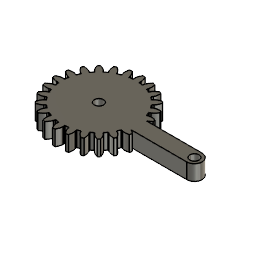
Simple gripper_Gear24 (Autodesk Fusion 360 design; units mm, degrees)
description: Spur Gear; Module: 1.125000; Num Teeth: 24; Pressure Angle: 20.000000; Backlash: 0.00 mm
Autodesk Fusion 360 part; units mm, degrees
(part 1 of 3)
sketch "Sketch4" plane through (0, 0, 3) normal (0, 0, 1) x (-1, 0, 0)
  arc A0 (-106.7629, 26.1027) -> (-106.8965, 25.0883) centre (-94.8448, 24.0176) ccw
  arc A1 (-107.004, 24.9974) -> (-106.8965, 25.0883) centre (-106.9961, 25.0971) ccw
  line L0 (-107.004, 24.9974) -> (-107.4897, 25.0359)
  spline S0 degree 5 poles (-107.4897, 25.0359) (-107.4953, 25.0363) (-107.5066, 25.0371) (-107.5235, 25.0378) (-107.5461, 25.0379) (-107.5744, 25.0371) (-107.6028, 25.0354) (-107.6311, 25.0332) (-107.6595, 25.0307) (-107.6879, 25.0281) (-107.7163, 25.0252) (-107.7447, 25.0221) (-107.7731, 25.0187) (-107.8015, 25.0149) (-107.83, 25.0108) (-107.8584, 25.0062) (-107.8868, 25.0014) (-107.9153, 24.9963) (-107.9437, 24.9909) (-107.9722, 24.9854) (-108.0006, 24.9796) (-108.029, 24.9736) (-108.0575, 24.9674) (-108.0859, 24.9609) (-108.1143, 24.9542) (-108.1428, 24.9473) (-108.1712, 24.9402) (-108.1996, 24.9328) (-108.228, 24.9252) (-108.2564, 24.9175) (-108.2848, 24.9095) (-108.3132, 24.9014) (-108.3416, 24.893) (-108.3699, 24.8845) (-108.3983, 24.8757) (-108.4266, 24.8668) (-108.455, 24.8577) (-108.4833, 24.8484) (-108.5116, 24.839) (-108.5399, 24.8293) (-108.5682, 24.8195) (-108.5965, 24.8095) (-108.6247, 24.7993) (-108.653, 24.789) (-108.6812, 24.7785) (-108.7094, 24.7678) (-108.7376, 24.7569) (-108.7658, 24.7459) (-108.794, 24.7347) (-108.8221, 24.7234) (-108.8503, 24.7119) (-108.8784, 24.7002) (-108.9065, 24.6884) (-108.9346, 24.6764) (-108.9627, 24.6643) (-108.9907, 24.652) (-109.0187, 24.6395) (-109.0467, 24.6269) (-109.0747, 24.6142) (-109.1027, 24.6013) (-109.1306, 24.5882) (-109.1586, 24.575) (-109.1865, 24.5616) (-109.2143, 24.5481) (-109.2422, 24.5345) (-109.27, 24.5207) (-109.2979, 24.5067) (-109.3256, 24.4927) (-109.3534, 24.4784) (-109.3811, 24.4641) (-109.4089, 24.4495) (-109.431, 24.4378) (-109.4476, 24.429) (-109.4587, 24.423) (-109.4642, 24.42) knots 0 0 0 0 0 0 0.01428571 0.02857143 0.04285714 0.05714286 0.07142857 0.08571429 0.1 0.11428571 0.12857143 0.14285714 0.15714286 0.17142857 0.18571429 0.2 0.21428571 0.22857143 0.24285714 0.25714286 0.27142857 0.28571429 0.3 0.31428571 0.32857143 0.34285714 0.35714286 0.37142857 0.38571429 0.4 0.41428571 0.42857143 0.44285714 0.45714286 0.47142857 0.48571429 0.5 0.51428571 0.52857143 0.54285714 0.55714286 0.57142857 0.58571429 0.6 0.61428571 0.62857143 0.64285714 0.65714286 0.67142857 0.68571429 0.7 0.71428571 0.72857143 0.74285714 0.75714286 0.77142857 0.78571429 0.8 0.81428571 0.82857143 0.84285714 0.85714286 0.87142857 0.88571429 0.9 0.91428571 0.92857143 0.94285714 0.95714286 0.97142857 0.98571429 1 1 1 1 1 1
  arc A2 (-109.4642, 24.42) -> (-109.4642, 23.6152) centre (-94.8448, 24.0176) ccw
  spline S1 degree 5 poles (-109.4642, 23.6152) (-109.4587, 23.6122) (-109.4476, 23.6062) (-109.431, 23.5974) (-109.4089, 23.5857) (-109.3811, 23.5712) (-109.3534, 23.5568) (-109.3256, 23.5425) (-109.2979, 23.5285) (-109.27, 23.5145) (-109.2422, 23.5007) (-109.2143, 23.4871) (-109.1865, 23.4736) (-109.1586, 23.4602) (-109.1306, 23.447) (-109.1027, 23.4339) (-109.0747, 23.421) (-109.0467, 23.4083) (-109.0187, 23.3957) (-108.9907, 23.3832) (-108.9627, 23.3709) (-108.9346, 23.3588) (-108.9065, 23.3468) (-108.8784, 23.335) (-108.8503, 23.3233) (-108.8221, 23.3118) (-108.794, 23.3005) (-108.7658, 23.2893) (-108.7376, 23.2783) (-108.7094, 23.2674) (-108.6812, 23.2568) (-108.653, 23.2462) (-108.6247, 23.2359) (-108.5965, 23.2257) (-108.5682, 23.2157) (-108.5399, 23.2059) (-108.5116, 23.1962) (-108.4833, 23.1868) (-108.455, 23.1775) (-108.4266, 23.1684) (-108.3983, 23.1595) (-108.3699, 23.1507) (-108.3416, 23.1422) (-108.3132, 23.1338) (-108.2848, 23.1257) (-108.2564, 23.1177) (-108.228, 23.11) (-108.1996, 23.1024) (-108.1712, 23.0951) (-108.1428, 23.0879) (-108.1143, 23.081) (-108.0859, 23.0743) (-108.0575, 23.0678) (-108.029, 23.0616) (-108.0006, 23.0556) (-107.9722, 23.0498) (-107.9437, 23.0443) (-107.9153, 23.0389) (-107.8868, 23.0338) (-107.8584, 23.029) (-107.83, 23.0244) (-107.8015, 23.0203) (-107.7731, 23.0165) (-107.7447, 23.0131) (-107.7163, 23.01) (-107.6879, 23.0071) (-107.6595, 23.0045) (-107.6311, 23.002) (-107.6028, 22.9998) (-107.5744, 22.9982) (-107.5461, 22.9973) (-107.5235, 22.9974) (-107.5066, 22.9981) (-107.4953, 22.9989) (-107.4897, 22.9993) knots -1 -1 -1 -1 -1 -1 -0.98571429 -0.97142857 -0.95714286 -0.94285714 -0.92857143 -0.91428571 -0.9 -0.88571429 -0.87142857 -0.85714286 -0.84285714 -0.82857143 -0.81428571 -0.8 -0.78571429 -0.77142857 -0.75714286 -0.74285714 -0.72857143 -0.71428571 -0.7 -0.68571429 -0.67142857 -0.65714286 -0.64285714 -0.62857143 -0.61428571 -0.6 -0.58571429 -0.57142857 -0.55714286 -0.54285714 -0.52857143 -0.51428571 -0.5 -0.48571429 -0.47142857 -0.45714286 -0.44285714 -0.42857143 -0.41428571 -0.4 -0.38571429 -0.37142857 -0.35714286 -0.34285714 -0.32857143 -0.31428571 -0.3 -0.28571429 -0.27142857 -0.25714286 -0.24285714 -0.22857143 -0.21428571 -0.2 -0.18571429 -0.17142857 -0.15714286 -0.14285714 -0.12857143 -0.11428571 -0.1 -0.08571429 -0.07142857 -0.05714286 -0.04285714 -0.02857143 -0.01428571 0 0 0 0 0 0
  line L1 (-107.4897, 22.9993) -> (-107.004, 23.0378)
  arc A3 (-106.8965, 22.947) -> (-107.004, 23.0378) centre (-106.9961, 22.9381) ccw
  arc A4 (-106.8965, 22.947) -> (-106.7629, 21.9326) centre (-94.8448, 24.0176) ccw
  arc A5 (-106.8433, 21.817) -> (-106.7629, 21.9326) centre (-106.8614, 21.9153) ccw
  line L2 (-106.8433, 21.817) -> (-107.3224, 21.7284)
  spline S2 degree 5 poles (-107.3224, 21.7284) (-107.3279, 21.7274) (-107.339, 21.7252) (-107.3556, 21.7215) (-107.3774, 21.7158) (-107.4045, 21.7076) (-107.4315, 21.6987) (-107.4583, 21.6892) (-107.4851, 21.6795) (-107.5118, 21.6696) (-107.5385, 21.6595) (-107.5651, 21.6492) (-107.5917, 21.6385) (-107.6182, 21.6275) (-107.6446, 21.6161) (-107.6709, 21.6044) (-107.6971, 21.5923) (-107.7232, 21.58) (-107.7493, 21.5675) (-107.7753, 21.5548) (-107.8013, 21.5418) (-107.8272, 21.5287) (-107.8531, 21.5153) (-107.8789, 21.5017) (-107.9046, 21.4879) (-107.9303, 21.4738) (-107.9559, 21.4596) (-107.9814, 21.4451) (-108.0069, 21.4305) (-108.0323, 21.4156) (-108.0577, 21.4006) (-108.083, 21.3854) (-108.1082, 21.37) (-108.1334, 21.3544) (-108.1586, 21.3386) (-108.1836, 21.3226) (-108.2086, 21.3065) (-108.2336, 21.2902) (-108.2585, 21.2737) (-108.2833, 21.2571) (-108.3081, 21.2403) (-108.3328, 21.2233) (-108.3575, 21.2062) (-108.3821, 21.1889) (-108.4067, 21.1714) (-108.4312, 21.1538) (-108.4556, 21.136) (-108.48, 21.118) (-108.5043, 21.1) (-108.5285, 21.0817) (-108.5527, 21.0633) (-108.5769, 21.0448) (-108.601, 21.0261) (-108.625, 21.0072) (-108.649, 20.9882) (-108.6729, 20.9691) (-108.6967, 20.9498) (-108.7205, 20.9304) (-108.7443, 20.9108) (-108.7679, 20.8911) (-108.7915, 20.8713) (-108.8151, 20.8513) (-108.8386, 20.8312) (-108.862, 20.8109) (-108.8854, 20.7905) (-108.9087, 20.77) (-108.932, 20.7493) (-108.9552, 20.7285) (-108.9783, 20.7076) (-109.0014, 20.6865) (-109.0244, 20.6654) (-109.0428, 20.6483) (-109.0565, 20.6354) (-109.0657, 20.6268) (-109.0702, 20.6225) knots 0 0 0 0 0 0 0.01428571 0.02857143 0.04285714 0.05714286 0.07142857 0.08571429 0.1 0.11428571 0.12857143 0.14285714 0.15714286 0.17142857 0.18571429 0.2 0.21428571 0.22857143 0.24285714 0.25714286 0.27142857 0.28571429 0.3 0.31428571 0.32857143 0.34285714 0.35714286 0.37142857 0.38571429 0.4 0.41428571 0.42857143 0.44285714 0.45714286 0.47142857 0.48571429 0.5 0.51428571 0.52857143 0.54285714 0.55714286 0.57142857 0.58571429 0.6 0.61428571 0.62857143 0.64285714 0.65714286 0.67142857 0.68571429 0.7 0.71428571 0.72857143 0.74285714 0.75714286 0.77142857 0.78571429 0.8 0.81428571 0.82857143 0.84285714 0.85714286 0.87142857 0.88571429 0.9 0.91428571 0.92857143 0.94285714 0.95714286 0.97142857 0.98571429 1 1 1 1 1 1
  arc A6 (-109.0702, 20.6225) -> (-108.8619, 19.8451) centre (-94.8448, 24.0176) ccw
  spline S3 degree 5 poles (-108.8619, 19.8451) (-108.8558, 19.8436) (-108.8436, 19.8408) (-108.8252, 19.8365) (-108.8008, 19.8309) (-108.7703, 19.8241) (-108.7398, 19.8174) (-108.7093, 19.8108) (-108.6788, 19.8044) (-108.6483, 19.7981) (-108.6178, 19.792) (-108.5874, 19.786) (-108.557, 19.7802) (-108.5266, 19.7745) (-108.4962, 19.769) (-108.4658, 19.7636) (-108.4354, 19.7584) (-108.4051, 19.7533) (-108.3748, 19.7484) (-108.3445, 19.7436) (-108.3142, 19.739) (-108.284, 19.7345) (-108.2538, 19.7302) (-108.2235, 19.7261) (-108.1934, 19.7221) (-108.1632, 19.7183) (-108.1331, 19.7146) (-108.103, 19.7111) (-108.0729, 19.7077) (-108.0428, 19.7046) (-108.0128, 19.7015) (-107.9828, 19.6987) (-107.9529, 19.696) (-107.9229, 19.6935) (-107.893, 19.6912) (-107.8632, 19.689) (-107.8333, 19.687) (-107.8035, 19.6852) (-107.7738, 19.6835) (-107.744, 19.6821) (-107.7144, 19.6808) (-107.6847, 19.6797) (-107.6551, 19.6788) (-107.6255, 19.6781) (-107.596, 19.6775) (-107.5665, 19.6772) (-107.5371, 19.6771) (-107.5077, 19.6771) (-107.4783, 19.6774) (-107.449, 19.6778) (-107.4198, 19.6785) (-107.3906, 19.6793) (-107.3614, 19.6805) (-107.3324, 19.6818) (-107.3033, 19.6834) (-107.2744, 19.6852) (-107.2455, 19.6872) (-107.2166, 19.6894) (-107.1878, 19.6918) (-107.1591, 19.6945) (-107.1305, 19.6975) (-107.1019, 19.7008) (-107.0735, 19.7045) (-107.0452, 19.7085) (-107.0169, 19.7129) (-106.9887, 19.7175) (-106.9606, 19.7223) (-106.9326, 19.7273) (-106.9046, 19.7325) (-106.8768, 19.7382) (-106.8493, 19.7447) (-106.8275, 19.7507) (-106.8113, 19.7557) (-106.8006, 19.7594) (-106.7953, 19.7613) knots -1 -1 -1 -1 -1 -1 -0.98571429 -0.97142857 -0.95714286 -0.94285714 -0.92857143 -0.91428571 -0.9 -0.88571429 -0.87142857 -0.85714286 -0.84285714 -0.82857143 -0.81428571 -0.8 -0.78571429 -0.77142857 -0.75714286 -0.74285714 -0.72857143 -0.71428571 -0.7 -0.68571429 -0.67142857 -0.65714286 -0.64285714 -0.62857143 -0.61428571 -0.6 -0.58571429 -0.57142857 -0.55714286 -0.54285714 -0.52857143 -0.51428571 -0.5 -0.48571429 -0.47142857 -0.45714286 -0.44285714 -0.42857143 -0.41428571 -0.4 -0.38571429 -0.37142857 -0.35714286 -0.34285714 -0.32857143 -0.31428571 -0.3 -0.28571429 -0.27142857 -0.25714286 -0.24285714 -0.22857143 -0.21428571 -0.2 -0.18571429 -0.17142857 -0.15714286 -0.14285714 -0.12857143 -0.11428571 -0.1 -0.08571429 -0.07142857 -0.05714286 -0.04285714 -0.02857143 -0.01428571 0 0 0 0 0 0
  line L3 (-106.7953, 19.7613) -> (-106.3361, 19.9241)
  arc A7 (-106.2087, 19.8642) -> (-106.3361, 19.9241) centre (-106.3027, 19.8299) ccw
  arc A8 (-106.2087, 19.8642) -> (-105.8172, 18.9189) centre (-94.8448, 24.0176) ccw
  arc A9 (-105.8649, 18.7865) -> (-105.8172, 18.9189) centre (-105.9079, 18.8768) ccw
  line L4 (-105.8649, 18.7865) -> (-106.3047, 18.577)
  spline S4 degree 5 poles (-106.3047, 18.577) (-106.3098, 18.5746) (-106.32, 18.5696) (-106.335, 18.5617) (-106.3546, 18.5505) (-106.3787, 18.5356) (-106.4024, 18.52) (-106.4259, 18.5039) (-106.4492, 18.4876) (-106.4725, 18.4711) (-106.4956, 18.4545) (-106.5187, 18.4376) (-106.5416, 18.4204) (-106.5643, 18.4029) (-106.5869, 18.3851) (-106.6092, 18.3669) (-106.6314, 18.3485) (-106.6535, 18.3299) (-106.6755, 18.311) (-106.6973, 18.292) (-106.7191, 18.2728) (-106.7407, 18.2534) (-106.7622, 18.2338) (-106.7836, 18.214) (-106.8049, 18.194) (-106.826, 18.1737) (-106.8471, 18.1533) (-106.868, 18.1328) (-106.8888, 18.112) (-106.9095, 18.0911) (-106.9301, 18.07) (-106.9506, 18.0487) (-106.971, 18.0273) (-106.9913, 18.0058) (-107.0115, 17.984) (-107.0316, 17.9621) (-107.0516, 17.9401) (-107.0715, 17.9178) (-107.0913, 17.8955) (-107.111, 17.873) (-107.1305, 17.8503) (-107.15, 17.8275) (-107.1694, 17.8046) (-107.1887, 17.7815) (-107.2079, 17.7583) (-107.227, 17.7349) (-107.246, 17.7114) (-107.2649, 17.6878) (-107.2837, 17.664) (-107.3024, 17.6401) (-107.321, 17.6161) (-107.3396, 17.5919) (-107.358, 17.5676) (-107.3763, 17.5432) (-107.3945, 17.5187) (-107.4127, 17.494) (-107.4307, 17.4692) (-107.4487, 17.4443) (-107.4666, 17.4193) (-107.4843, 17.3941) (-107.502, 17.3688) (-107.5196, 17.3434) (-107.5371, 17.3179) (-107.5544, 17.2923) (-107.5718, 17.2665) (-107.589, 17.2406) (-107.6061, 17.2147) (-107.6231, 17.1886) (-107.64, 17.1624) (-107.6569, 17.136) (-107.6736, 17.1096) (-107.6869, 17.0884) (-107.6969, 17.0724) (-107.7035, 17.0617) (-107.7068, 17.0564) knots 0 0 0 0 0 0 0.01428571 0.02857143 0.04285714 0.05714286 0.07142857 0.08571429 0.1 0.11428571 0.12857143 0.14285714 0.15714286 0.17142857 0.18571429 0.2 0.21428571 0.22857143 0.24285714 0.25714286 0.27142857 0.28571429 0.3 0.31428571 0.32857143 0.34285714 0.35714286 0.37142857 0.38571429 0.4 0.41428571 0.42857143 0.44285714 0.45714286 0.47142857 0.48571429 0.5 0.51428571 0.52857143 0.54285714 0.55714286 0.57142857 0.58571429 0.6 0.61428571 0.62857143 0.64285714 0.65714286 0.67142857 0.68571429 0.7 0.71428571 0.72857143 0.74285714 0.75714286 0.77142857 0.78571429 0.8 0.81428571 0.82857143 0.84285714 0.85714286 0.87142857 0.88571429 0.9 0.91428571 0.92857143 0.94285714 0.95714286 0.97142857 0.98571429 1 1 1 1 1 1
  arc A10 (-107.7068, 17.0564) -> (-107.3044, 16.3593) centre (-94.8448, 24.0176) ccw
  spline S5 degree 5 poles (-107.3044, 16.3593) (-107.2981, 16.3595) (-107.2855, 16.3599) (-107.2667, 16.3606) (-107.2417, 16.3615) (-107.2104, 16.3628) (-107.1792, 16.3642) (-107.148, 16.3657) (-107.1169, 16.3674) (-107.0859, 16.3693) (-107.0549, 16.3712) (-107.0239, 16.3734) (-106.993, 16.3756) (-106.9622, 16.378) (-106.9314, 16.3805) (-106.9007, 16.3832) (-106.87, 16.386) (-106.8394, 16.3889) (-106.8088, 16.392) (-106.7783, 16.3952) (-106.7479, 16.3986) (-106.7175, 16.4021) (-106.6872, 16.4058) (-106.6569, 16.4096) (-106.6268, 16.4136) (-106.5966, 16.4177) (-106.5666, 16.4219) (-106.5366, 16.4263) (-106.5067, 16.4309) (-106.4768, 16.4356) (-106.4471, 16.4405) (-106.4173, 16.4455) (-106.3877, 16.4506) (-106.3581, 16.456) (-106.3287, 16.4614) (-106.2993, 16.4671) (-106.2699, 16.4729) (-106.2407, 16.4788) (-106.2115, 16.4849) (-106.1824, 16.4912) (-106.1534, 16.4977) (-106.1245, 16.5043) (-106.0956, 16.5111) (-106.0669, 16.518) (-106.0382, 16.5252) (-106.0097, 16.5325) (-105.9812, 16.5399) (-105.9528, 16.5476) (-105.9245, 16.5554) (-105.8963, 16.5634) (-105.8682, 16.5717) (-105.8403, 16.5801) (-105.8124, 16.5887) (-105.7847, 16.5975) (-105.7571, 16.6066) (-105.7295, 16.6158) (-105.7021, 16.6252) (-105.6748, 16.6348) (-105.6477, 16.6446) (-105.6206, 16.6546) (-105.5937, 16.6649) (-105.567, 16.6755) (-105.5405, 16.6864) (-105.5142, 16.6977) (-105.488, 16.7092) (-105.462, 16.7209) (-105.4361, 16.7328) (-105.4103, 16.7449) (-105.3846, 16.7572) (-105.3593, 16.7699) (-105.3343, 16.7833) (-105.3148, 16.7947) (-105.3005, 16.8038) (-105.2911, 16.8101) (-105.2864, 16.8133) knots -1 -1 -1 -1 -1 -1 -0.98571429 -0.97142857 -0.95714286 -0.94285714 -0.92857143 -0.91428571 -0.9 -0.88571429 -0.87142857 -0.85714286 -0.84285714 -0.82857143 -0.81428571 -0.8 -0.78571429 -0.77142857 -0.75714286 -0.74285714 -0.72857143 -0.71428571 -0.7 -0.68571429 -0.67142857 -0.65714286 -0.64285714 -0.62857143 -0.61428571 -0.6 -0.58571429 -0.57142857 -0.55714286 -0.54285714 -0.52857143 -0.51428571 -0.5 -0.48571429 -0.47142857 -0.45714286 -0.44285714 -0.42857143 -0.41428571 -0.4 -0.38571429 -0.37142857 -0.35714286 -0.34285714 -0.32857143 -0.31428571 -0.3 -0.28571429 -0.27142857 -0.25714286 -0.24285714 -0.22857143 -0.21428571 -0.2 -0.18571429 -0.17142857 -0.15714286 -0.14285714 -0.12857143 -0.11428571 -0.1 -0.08571429 -0.07142857 -0.05714286 -0.04285714 -0.02857143 -0.01428571 0 0 0 0 0 0
  line L5 (-105.2864, 16.8133) -> (-104.8851, 17.0894)
  arc A11 (-104.7465, 17.0645) -> (-104.8851, 17.0894) centre (-104.8284, 17.0071) ccw
  arc A12 (-104.7465, 17.0645) -> (-104.1237, 16.2528) centre (-94.8448, 24.0176) ccw
  arc A13 (-104.1355, 16.1126) -> (-104.1237, 16.2528) centre (-104.2004, 16.1886) ccw
  line L6 (-104.1355, 16.1126) -> (-104.5061, 15.7963)
  spline S6 degree 5 poles (-104.5061, 15.7963) (-104.5104, 15.7926) (-104.5189, 15.7852) (-104.5314, 15.7737) (-104.5475, 15.7579) (-104.5669, 15.7372) (-104.5857, 15.716) (-104.6042, 15.6944) (-104.6225, 15.6726) (-104.6407, 15.6506) (-104.6588, 15.6286) (-104.6767, 15.6063) (-104.6944, 15.5838) (-104.7118, 15.561) (-104.729, 15.5379) (-104.7459, 15.5146) (-104.7625, 15.4911) (-104.779, 15.4674) (-104.7954, 15.4435) (-104.8116, 15.4194) (-104.8276, 15.3952) (-104.8435, 15.3709) (-104.8592, 15.3464) (-104.8747, 15.3217) (-104.8901, 15.2969) (-104.9053, 15.2719) (-104.9203, 15.2467) (-104.9352, 15.2214) (-104.9499, 15.196) (-104.9645, 15.1704) (-104.979, 15.1447) (-104.9933, 15.1189) (-105.0075, 15.0929) (-105.0215, 15.0668) (-105.0353, 15.0406) (-105.0491, 15.0143) (-105.0627, 14.9878) (-105.0761, 14.9612) (-105.0895, 14.9345) (-105.1027, 14.9076) (-105.1157, 14.8807) (-105.1286, 14.8536) (-105.1414, 14.8264) (-105.1541, 14.7992) (-105.1666, 14.7718) (-105.179, 14.7442) (-105.1913, 14.7166) (-105.2034, 14.6889) (-105.2154, 14.6611) (-105.2273, 14.6332) (-105.2391, 14.6051) (-105.2507, 14.577) (-105.2622, 14.5488) (-105.2736, 14.5204) (-105.2849, 14.492) (-105.296, 14.4635) (-105.307, 14.4348) (-105.3179, 14.4061) (-105.3287, 14.3773) (-105.3393, 14.3484) (-105.3499, 14.3194) (-105.3603, 14.2903) (-105.3706, 14.2612) (-105.3807, 14.2319) (-105.3908, 14.2026) (-105.4007, 14.1731) (-105.4105, 14.1436) (-105.4202, 14.114) (-105.4298, 14.0843) (-105.4392, 14.0545) (-105.4486, 14.0246) (-105.4559, 14.0007) (-105.4614, 13.9827) (-105.465, 13.9707) (-105.4668, 13.9647) knots 0 0 0 0 0 0 0.01428571 0.02857143 0.04285714 0.05714286 0.07142857 0.08571429 0.1 0.11428571 0.12857143 0.14285714 0.15714286 0.17142857 0.18571429 0.2 0.21428571 0.22857143 0.24285714 0.25714286 0.27142857 0.28571429 0.3 0.31428571 0.32857143 0.34285714 0.35714286 0.37142857 0.38571429 0.4 0.41428571 0.42857143 0.44285714 0.45714286 0.47142857 0.48571429 0.5 0.51428571 0.52857143 0.54285714 0.55714286 0.57142857 0.58571429 0.6 0.61428571 0.62857143 0.64285714 0.65714286 0.67142857 0.68571429 0.7 0.71428571 0.72857143 0.74285714 0.75714286 0.77142857 0.78571429 0.8 0.81428571 0.82857143 0.84285714 0.85714286 0.87142857 0.88571429 0.9 0.91428571 0.92857143 0.94285714 0.95714286 0.97142857 0.98571429 1 1 1 1 1 1
  arc A14 (-105.4668, 13.9647) -> (-104.8977, 13.3955) centre (-94.8448, 24.0176) ccw
  spline S7 degree 5 poles (-104.8977, 13.3955) (-104.8917, 13.3973) (-104.8797, 13.4009) (-104.8617, 13.4064) (-104.8377, 13.4138) (-104.8078, 13.4231) (-104.7781, 13.4326) (-104.7484, 13.4422) (-104.7188, 13.4518) (-104.6892, 13.4617) (-104.6598, 13.4716) (-104.6304, 13.4816) (-104.6012, 13.4918) (-104.572, 13.5021) (-104.5429, 13.5125) (-104.5139, 13.523) (-104.485, 13.5337) (-104.4562, 13.5444) (-104.4275, 13.5553) (-104.3989, 13.5663) (-104.3704, 13.5775) (-104.3419, 13.5887) (-104.3136, 13.6001) (-104.2854, 13.6116) (-104.2572, 13.6233) (-104.2292, 13.635) (-104.2013, 13.6469) (-104.1734, 13.6589) (-104.1457, 13.6711) (-104.1181, 13.6833) (-104.0906, 13.6957) (-104.0632, 13.7083) (-104.0359, 13.7209) (-104.0087, 13.7337) (-103.9817, 13.7466) (-103.9547, 13.7597) (-103.9279, 13.7729) (-103.9012, 13.7862) (-103.8746, 13.7997) (-103.8481, 13.8133) (-103.8217, 13.827) (-103.7955, 13.8409) (-103.7694, 13.8549) (-103.7435, 13.8691) (-103.7176, 13.8834) (-103.6919, 13.8978) (-103.6664, 13.9124) (-103.6409, 13.9272) (-103.6156, 13.942) (-103.5905, 13.9571) (-103.5655, 13.9723) (-103.5406, 13.9876) (-103.516, 14.0032) (-103.4914, 14.0189) (-103.4671, 14.0348) (-103.4429, 14.0508) (-103.4189, 14.067) (-103.395, 14.0833) (-103.3713, 14.0998) (-103.3477, 14.1165) (-103.3244, 14.1334) (-103.3014, 14.1505) (-103.2786, 14.168) (-103.2561, 14.1856) (-103.2338, 14.2035) (-103.2117, 14.2216) (-103.1898, 14.2398) (-103.168, 14.2581) (-103.1464, 14.2767) (-103.1251, 14.2955) (-103.1045, 14.3149) (-103.0886, 14.331) (-103.0772, 14.3435) (-103.0697, 14.352) (-103.066, 14.3563) knots -1 -1 -1 -1 -1 -1 -0.98571429 -0.97142857 -0.95714286 -0.94285714 -0.92857143 -0.91428571 -0.9 -0.88571429 -0.87142857 -0.85714286 -0.84285714 -0.82857143 -0.81428571 -0.8 -0.78571429 -0.77142857 -0.75714286 -0.74285714 -0.72857143 -0.71428571 -0.7 -0.68571429 -0.67142857 -0.65714286 -0.64285714 -0.62857143 -0.61428571 -0.6 -0.58571429 -0.57142857 -0.55714286 -0.54285714 -0.52857143 -0.51428571 -0.5 -0.48571429 -0.47142857 -0.45714286 -0.44285714 -0.42857143 -0.41428571 -0.4 -0.38571429 -0.37142857 -0.35714286 -0.34285714 -0.32857143 -0.31428571 -0.3 -0.28571429 -0.27142857 -0.25714286 -0.24285714 -0.22857143 -0.21428571 -0.2 -0.18571429 -0.17142857 -0.15714286 -0.14285714 -0.12857143 -0.11428571 -0.1 -0.08571429 -0.07142857 -0.05714286 -0.04285714 -0.02857143 -0.01428571 0 0 0 0 0 0
  line L7 (-103.066, 14.3563) -> (-102.7498, 14.7269)
  arc A15 (-102.6096, 14.7387) -> (-102.7498, 14.7269) centre (-102.6737, 14.662) ccw
  arc A16 (-102.6096, 14.7387) -> (-101.7978, 14.1158) centre (-94.8448, 24.0176) ccw
  arc A17 (-101.7729, 13.9773) -> (-101.7978, 14.1158) centre (-101.8553, 14.034) ccw
  line L8 (-101.7729, 13.9773) -> (-102.0491, 13.5759)
  spline S8 degree 5 poles (-102.0491, 13.5759) (-102.0523, 13.5713) (-102.0586, 13.5619) (-102.0676, 13.5475) (-102.0791, 13.528) (-102.0925, 13.5031) (-102.1052, 13.4777) (-102.1175, 13.4521) (-102.1295, 13.4263) (-102.1414, 13.4004) (-102.1532, 13.3743) (-102.1647, 13.3482) (-102.1759, 13.3219) (-102.1869, 13.2954) (-102.1975, 13.2686) (-102.2077, 13.2418) (-102.2178, 13.2147) (-102.2276, 13.1875) (-102.2372, 13.1602) (-102.2466, 13.1328) (-102.2558, 13.1053) (-102.2648, 13.0777) (-102.2737, 13.0499) (-102.2823, 13.0221) (-102.2907, 12.9941) (-102.2989, 12.966) (-102.3069, 12.9378) (-102.3148, 12.9096) (-102.3224, 12.8812) (-102.3299, 12.8527) (-102.3372, 12.8241) (-102.3443, 12.7955) (-102.3513, 12.7667) (-102.3581, 12.7379) (-102.3647, 12.709) (-102.3711, 12.68) (-102.3774, 12.6509) (-102.3835, 12.6217) (-102.3895, 12.5924) (-102.3953, 12.5631) (-102.4009, 12.5337) (-102.4064, 12.5042) (-102.4117, 12.4746) (-102.4169, 12.445) (-102.4219, 12.4153) (-102.4268, 12.3855) (-102.4315, 12.3557) (-102.436, 12.3258) (-102.4404, 12.2958) (-102.4447, 12.2657) (-102.4488, 12.2356) (-102.4527, 12.2054) (-102.4565, 12.1752) (-102.4602, 12.1448) (-102.4637, 12.1145) (-102.4671, 12.084) (-102.4703, 12.0535) (-102.4734, 12.023) (-102.4764, 11.9924) (-102.4792, 11.9617) (-102.4818, 11.931) (-102.4844, 11.9002) (-102.4868, 11.8693) (-102.489, 11.8384) (-102.4911, 11.8075) (-102.4931, 11.7765) (-102.4949, 11.7454) (-102.4966, 11.7143) (-102.4982, 11.6832) (-102.4996, 11.6519) (-102.5009, 11.6207) (-102.5018, 11.5956) (-102.5024, 11.5768) (-102.5028, 11.5643) (-102.503, 11.558) knots 0 0 0 0 0 0 0.01428571 0.02857143 0.04285714 0.05714286 0.07142857 0.08571429 0.1 0.11428571 0.12857143 0.14285714 0.15714286 0.17142857 0.18571429 0.2 0.21428571 0.22857143 0.24285714 0.25714286 0.27142857 0.28571429 0.3 0.31428571 0.32857143 0.34285714 0.35714286 0.37142857 0.38571429 0.4 0.41428571 0.42857143 0.44285714 0.45714286 0.47142857 0.48571429 0.5 0.51428571 0.52857143 0.54285714 0.55714286 0.57142857 0.58571429 0.6 0.61428571 0.62857143 0.64285714 0.65714286 0.67142857 0.68571429 0.7 0.71428571 0.72857143 0.74285714 0.75714286 0.77142857 0.78571429 0.8 0.81428571 0.82857143 0.84285714 0.85714286 0.87142857 0.88571429 0.9 0.91428571 0.92857143 0.94285714 0.95714286 0.97142857 0.98571429 1 1 1 1 1 1
  arc A18 (-102.503, 11.558) -> (-101.806, 11.1556) centre (-94.8448, 24.0176) ccw
  spline S9 degree 5 poles (-101.806, 11.1556) (-101.8006, 11.1589) (-101.7899, 11.1655) (-101.774, 11.1754) (-101.7527, 11.1887) (-101.7263, 11.2055) (-101.7, 11.2223) (-101.6738, 11.2393) (-101.6477, 11.2563) (-101.6217, 11.2734) (-101.5958, 11.2906) (-101.5701, 11.3079) (-101.5445, 11.3253) (-101.5189, 11.3428) (-101.4935, 11.3604) (-101.4683, 11.378) (-101.4431, 11.3958) (-101.4181, 11.4137) (-101.3931, 11.4316) (-101.3683, 11.4497) (-101.3437, 11.4678) (-101.3191, 11.486) (-101.2947, 11.5044) (-101.2704, 11.5228) (-101.2463, 11.5413) (-101.2222, 11.5599) (-101.1983, 11.5786) (-101.1746, 11.5975) (-101.1509, 11.6164) (-101.1274, 11.6354) (-101.1041, 11.6545) (-101.0808, 11.6736) (-101.0578, 11.6929) (-101.0348, 11.7123) (-101.012, 11.7318) (-100.9894, 11.7514) (-100.9669, 11.7711) (-100.9445, 11.7909) (-100.9223, 11.8108) (-100.9002, 11.8307) (-100.8783, 11.8508) (-100.8566, 11.871) (-100.835, 11.8913) (-100.8136, 11.9117) (-100.7924, 11.9322) (-100.7713, 11.9528) (-100.7504, 11.9735) (-100.7296, 11.9944) (-100.709, 12.0153) (-100.6886, 12.0363) (-100.6684, 12.0575) (-100.6484, 12.0788) (-100.6286, 12.1001) (-100.609, 12.1217) (-100.5896, 12.1433) (-100.5703, 12.165) (-100.5513, 12.1869) (-100.5325, 12.2089) (-100.5138, 12.2309) (-100.4954, 12.2531) (-100.4773, 12.2755) (-100.4594, 12.298) (-100.4419, 12.3207) (-100.4248, 12.3436) (-100.4079, 12.3667) (-100.3912, 12.3899) (-100.3747, 12.4131) (-100.3584, 12.4365) (-100.3423, 12.4599) (-100.3267, 12.4836) (-100.3118, 12.5077) (-100.3006, 12.5274) (-100.2928, 12.5424) (-100.2878, 12.5525) (-100.2854, 12.5577) knots -1 -1 -1 -1 -1 -1 -0.98571429 -0.97142857 -0.95714286 -0.94285714 -0.92857143 -0.91428571 -0.9 -0.88571429 -0.87142857 -0.85714286 -0.84285714 -0.82857143 -0.81428571 -0.8 -0.78571429 -0.77142857 -0.75714286 -0.74285714 -0.72857143 -0.71428571 -0.7 -0.68571429 -0.67142857 -0.65714286 -0.64285714 -0.62857143 -0.61428571 -0.6 -0.58571429 -0.57142857 -0.55714286 -0.54285714 -0.52857143 -0.51428571 -0.5 -0.48571429 -0.47142857 -0.45714286 -0.44285714 -0.42857143 -0.41428571 -0.4 -0.38571429 -0.37142857 -0.35714286 -0.34285714 -0.32857143 -0.31428571 -0.3 -0.28571429 -0.27142857 -0.25714286 -0.24285714 -0.22857143 -0.21428571 -0.2 -0.18571429 -0.17142857 -0.15714286 -0.14285714 -0.12857143 -0.11428571 -0.1 -0.08571429 -0.07142857 -0.05714286 -0.04285714 -0.02857143 -0.01428571 0 0 0 0 0 0
  line L9 (-100.2854, 12.5577) -> (-100.0758, 12.9975)
  arc A19 (-99.9434, 13.0452) -> (-100.0758, 12.9975) centre (-99.9856, 12.9545) ccw
  arc A20 (-99.9434, 13.0452) -> (-98.9981, 12.6536) centre (-94.8448, 24.0176) ccw
  arc A21 (-98.9382, 12.5263) -> (-98.9981, 12.6536) centre (-99.0325, 12.5597) ccw
  line L10 (-98.9382, 12.5263) -> (-99.1011, 12.0671)
  spline S10 degree 5 poles (-99.1011, 12.0671) (-99.103, 12.0618) (-99.1066, 12.0511) (-99.1117, 12.0349) (-99.1177, 12.0131) (-99.1242, 11.9855) (-99.1299, 11.9577) (-99.1351, 11.9298) (-99.1401, 11.9017) (-99.1448, 11.8736) (-99.1494, 11.8454) (-99.1538, 11.8172) (-99.1579, 11.7889) (-99.1616, 11.7604) (-99.1649, 11.7319) (-99.1679, 11.7032) (-99.1705, 11.6745) (-99.173, 11.6457) (-99.1752, 11.6169) (-99.1772, 11.588) (-99.179, 11.559) (-99.1805, 11.53) (-99.1819, 11.5009) (-99.183, 11.4718) (-99.1839, 11.4426) (-99.1846, 11.4133) (-99.185, 11.384) (-99.1852, 11.3547) (-99.1853, 11.3253) (-99.1851, 11.2958) (-99.1848, 11.2664) (-99.1843, 11.2368) (-99.1836, 11.2073) (-99.1827, 11.1776) (-99.1816, 11.148) (-99.1803, 11.1183) (-99.1788, 11.0886) (-99.1772, 11.0588) (-99.1754, 11.029) (-99.1734, 10.9992) (-99.1712, 10.9693) (-99.1689, 10.9394) (-99.1663, 10.9095) (-99.1637, 10.8795) (-99.1608, 10.8495) (-99.1578, 10.8195) (-99.1546, 10.7895) (-99.1513, 10.7594) (-99.1478, 10.7293) (-99.1441, 10.6991) (-99.1403, 10.669) (-99.1363, 10.6388) (-99.1321, 10.6086) (-99.1278, 10.5784) (-99.1234, 10.5481) (-99.1187, 10.5178) (-99.114, 10.4876) (-99.1091, 10.4572) (-99.104, 10.4269) (-99.0987, 10.3966) (-99.0934, 10.3662) (-99.0878, 10.3358) (-99.0822, 10.3054) (-99.0763, 10.275) (-99.0704, 10.2445) (-99.0642, 10.2141) (-99.058, 10.1836) (-99.0515, 10.1531) (-99.045, 10.1226) (-99.0383, 10.0921) (-99.0314, 10.0615) (-99.0258, 10.0371) (-99.0216, 10.0188) (-99.0187, 10.0066) (-99.0173, 10.0004) knots 0 0 0 0 0 0 0.01428571 0.02857143 0.04285714 0.05714286 0.07142857 0.08571429 0.1 0.11428571 0.12857143 0.14285714 0.15714286 0.17142857 0.18571429 0.2 0.21428571 0.22857143 0.24285714 0.25714286 0.27142857 0.28571429 0.3 0.31428571 0.32857143 0.34285714 0.35714286 0.37142857 0.38571429 0.4 0.41428571 0.42857143 0.44285714 0.45714286 0.47142857 0.48571429 0.5 0.51428571 0.52857143 0.54285714 0.55714286 0.57142857 0.58571429 0.6 0.61428571 0.62857143 0.64285714 0.65714286 0.67142857 0.68571429 0.7 0.71428571 0.72857143 0.74285714 0.75714286 0.77142857 0.78571429 0.8 0.81428571 0.82857143 0.84285714 0.85714286 0.87142857 0.88571429 0.9 0.91428571 0.92857143 0.94285714 0.95714286 0.97142857 0.98571429 1 1 1 1 1 1
  arc A22 (-99.0173, 10.0004) -> (-98.2398, 9.7921) centre (-94.8448, 24.0176) ccw
  spline S11 degree 5 poles (-98.2398, 9.7921) (-98.2355, 9.7967) (-98.2269, 9.8059) (-98.2141, 9.8196) (-98.197, 9.838) (-98.1758, 9.861) (-98.1547, 9.8841) (-98.1338, 9.9072) (-98.113, 9.9304) (-98.0924, 9.9536) (-98.0718, 9.977) (-98.0514, 10.0003) (-98.0312, 10.0238) (-98.011, 10.0473) (-97.9911, 10.0708) (-97.9712, 10.0944) (-97.9515, 10.1181) (-97.9319, 10.1418) (-97.9125, 10.1656) (-97.8932, 10.1895) (-97.8741, 10.2134) (-97.8551, 10.2374) (-97.8363, 10.2614) (-97.8176, 10.2855) (-97.799, 10.3096) (-97.7806, 10.3338) (-97.7624, 10.3581) (-97.7443, 10.3824) (-97.7264, 10.4068) (-97.7086, 10.4312) (-97.691, 10.4557) (-97.6735, 10.4802) (-97.6562, 10.5048) (-97.6391, 10.5295) (-97.6221, 10.5542) (-97.6053, 10.579) (-97.5886, 10.6039) (-97.5722, 10.6288) (-97.5558, 10.6537) (-97.5397, 10.6787) (-97.5238, 10.7038) (-97.508, 10.7289) (-97.4924, 10.7541) (-97.477, 10.7794) (-97.4618, 10.8047) (-97.4467, 10.83) (-97.4319, 10.8555) (-97.4172, 10.8809) (-97.4028, 10.9065) (-97.3885, 10.9321) (-97.3745, 10.9577) (-97.3606, 10.9835) (-97.347, 11.0093) (-97.3337, 11.0351) (-97.3205, 11.061) (-97.3076, 11.087) (-97.2949, 11.1131) (-97.2823, 11.1391) (-97.27, 11.1653) (-97.258, 11.1915) (-97.2463, 11.2178) (-97.2349, 11.2442) (-97.2238, 11.2706) (-97.2132, 11.2972) (-97.2029, 11.3239) (-97.1928, 11.3506) (-97.1829, 11.3773) (-97.1731, 11.4041) (-97.1637, 11.4309) (-97.1547, 11.4578) (-97.1465, 11.4849) (-97.1408, 11.5068) (-97.1371, 11.5233) (-97.135, 11.5344) (-97.1339, 11.54) knots -1 -1 -1 -1 -1 -1 -0.98571429 -0.97142857 -0.95714286 -0.94285714 -0.92857143 -0.91428571 -0.9 -0.88571429 -0.87142857 -0.85714286 -0.84285714 -0.82857143 -0.81428571 -0.8 -0.78571429 -0.77142857 -0.75714286 -0.74285714 -0.72857143 -0.71428571 -0.7 -0.68571429 -0.67142857 -0.65714286 -0.64285714 -0.62857143 -0.61428571 -0.6 -0.58571429 -0.57142857 -0.55714286 -0.54285714 -0.52857143 -0.51428571 -0.5 -0.48571429 -0.47142857 -0.45714286 -0.44285714 -0.42857143 -0.41428571 -0.4 -0.38571429 -0.37142857 -0.35714286 -0.34285714 -0.32857143 -0.31428571 -0.3 -0.28571429 -0.27142857 -0.25714286 -0.24285714 -0.22857143 -0.21428571 -0.2 -0.18571429 -0.17142857 -0.15714286 -0.14285714 -0.12857143 -0.11428571 -0.1 -0.08571429 -0.07142857 -0.05714286 -0.04285714 -0.02857143 -0.01428571 0 0 0 0 0 0
  line L11 (-97.1339, 11.54) -> (-97.0454, 12.0191)
  arc A23 (-96.9298, 12.0994) -> (-97.0454, 12.0191) centre (-96.947, 12.0009) ccw
  arc A24 (-96.9298, 12.0994) -> (-95.9154, 11.9659) centre (-94.8448, 24.0176) ccw
  arc A25 (-95.8246, 11.8584) -> (-95.9154, 11.9659) centre (-95.9242, 11.8663) ccw
  line L12 (-95.8246, 11.8584) -> (-95.863, 11.3727)
  spline S12 degree 5 poles (-95.863, 11.3727) (-95.8635, 11.367) (-95.8642, 11.3558) (-95.8649, 11.3388) (-95.8651, 11.3162) (-95.8642, 11.2879) (-95.8625, 11.2596) (-95.8603, 11.2312) (-95.8579, 11.2029) (-95.8552, 11.1745) (-95.8524, 11.1461) (-95.8493, 11.1177) (-95.8459, 11.0892) (-95.8421, 11.0608) (-95.8379, 11.0324) (-95.8334, 11.0039) (-95.8285, 10.9755) (-95.8234, 10.9471) (-95.8181, 10.9186) (-95.8125, 10.8902) (-95.8068, 10.8617) (-95.8008, 10.8333) (-95.7945, 10.8049) (-95.7881, 10.7764) (-95.7814, 10.748) (-95.7745, 10.7196) (-95.7673, 10.6912) (-95.7599, 10.6628) (-95.7524, 10.6343) (-95.7446, 10.6059) (-95.7367, 10.5776) (-95.7285, 10.5492) (-95.7202, 10.5208) (-95.7116, 10.4924) (-95.7029, 10.4641) (-95.694, 10.4357) (-95.6849, 10.4074) (-95.6756, 10.3791) (-95.6661, 10.3507) (-95.6565, 10.3224) (-95.6466, 10.2942) (-95.6366, 10.2659) (-95.6265, 10.2376) (-95.6161, 10.2094) (-95.6056, 10.1811) (-95.5949, 10.1529) (-95.5841, 10.1247) (-95.5731, 10.0965) (-95.5619, 10.0684) (-95.5505, 10.0402) (-95.539, 10.0121) (-95.5274, 9.984) (-95.5155, 9.9558) (-95.5036, 9.9278) (-95.4914, 9.8997) (-95.4791, 9.8717) (-95.4667, 9.8436) (-95.4541, 9.8156) (-95.4413, 9.7876) (-95.4284, 9.7597) (-95.4153, 9.7317) (-95.4021, 9.7038) (-95.3888, 9.6759) (-95.3753, 9.648) (-95.3616, 9.6202) (-95.3478, 9.5923) (-95.3339, 9.5645) (-95.3198, 9.5367) (-95.3056, 9.509) (-95.2912, 9.4812) (-95.2767, 9.4535) (-95.265, 9.4313) (-95.2561, 9.4147) (-95.2502, 9.4037) (-95.2472, 9.3981) knots 0 0 0 0 0 0 0.01428571 0.02857143 0.04285714 0.05714286 0.07142857 0.08571429 0.1 0.11428571 0.12857143 0.14285714 0.15714286 0.17142857 0.18571429 0.2 0.21428571 0.22857143 0.24285714 0.25714286 0.27142857 0.28571429 0.3 0.31428571 0.32857143 0.34285714 0.35714286 0.37142857 0.38571429 0.4 0.41428571 0.42857143 0.44285714 0.45714286 0.47142857 0.48571429 0.5 0.51428571 0.52857143 0.54285714 0.55714286 0.57142857 0.58571429 0.6 0.61428571 0.62857143 0.64285714 0.65714286 0.67142857 0.68571429 0.7 0.71428571 0.72857143 0.74285714 0.75714286 0.77142857 0.78571429 0.8 0.81428571 0.82857143 0.84285714 0.85714286 0.87142857 0.88571429 0.9 0.91428571 0.92857143 0.94285714 0.95714286 0.97142857 0.98571429 1 1 1 1 1 1
  arc A26 (-95.2472, 9.3981) -> (-94.4423, 9.3981) centre (-94.8448, 24.0176) ccw
  spline S13 degree 5 poles (-94.4423, 9.3981) (-94.4393, 9.4037) (-94.4334, 9.4147) (-94.4245, 9.4313) (-94.4128, 9.4535) (-94.3983, 9.4812) (-94.3839, 9.509) (-94.3697, 9.5367) (-94.3556, 9.5645) (-94.3417, 9.5923) (-94.3279, 9.6202) (-94.3142, 9.648) (-94.3007, 9.6759) (-94.2874, 9.7038) (-94.2742, 9.7317) (-94.2611, 9.7597) (-94.2482, 9.7876) (-94.2354, 9.8156) (-94.2228, 9.8436) (-94.2104, 9.8717) (-94.1981, 9.8997) (-94.1859, 9.9278) (-94.174, 9.9558) (-94.1621, 9.984) (-94.1505, 10.0121) (-94.139, 10.0402) (-94.1276, 10.0684) (-94.1165, 10.0965) (-94.1054, 10.1247) (-94.0946, 10.1529) (-94.0839, 10.1811) (-94.0734, 10.2094) (-94.063, 10.2376) (-94.0529, 10.2659) (-94.0429, 10.2942) (-94.033, 10.3224) (-94.0234, 10.3507) (-94.0139, 10.3791) (-94.0046, 10.4074) (-93.9955, 10.4357) (-93.9866, 10.4641) (-93.9779, 10.4924) (-93.9693, 10.5208) (-93.961, 10.5492) (-93.9528, 10.5776) (-93.9449, 10.6059) (-93.9371, 10.6343) (-93.9296, 10.6628) (-93.9222, 10.6912) (-93.915, 10.7196) (-93.9081, 10.748) (-93.9014, 10.7764) (-93.895, 10.8049) (-93.8887, 10.8333) (-93.8827, 10.8617) (-93.877, 10.8902) (-93.8714, 10.9186) (-93.8661, 10.9471) (-93.861, 10.9755) (-93.8561, 11.0039) (-93.8516, 11.0324) (-93.8474, 11.0608) (-93.8436, 11.0892) (-93.8402, 11.1177) (-93.8371, 11.1461) (-93.8343, 11.1745) (-93.8316, 11.2029) (-93.8292, 11.2312) (-93.827, 11.2596) (-93.8253, 11.2879) (-93.8244, 11.3162) (-93.8246, 11.3388) (-93.8253, 11.3558) (-93.826, 11.367) (-93.8265, 11.3727) knots -1 -1 -1 -1 -1 -1 -0.98571429 -0.97142857 -0.95714286 -0.94285714 -0.92857143 -0.91428571 -0.9 -0.88571429 -0.87142857 -0.85714286 -0.84285714 -0.82857143 -0.81428571 -0.8 -0.78571429 -0.77142857 -0.75714286 -0.74285714 -0.72857143 -0.71428571 -0.7 -0.68571429 -0.67142857 -0.65714286 -0.64285714 -0.62857143 -0.61428571 -0.6 -0.58571429 -0.57142857 -0.55714286 -0.54285714 -0.52857143 -0.51428571 -0.5 -0.48571429 -0.47142857 -0.45714286 -0.44285714 -0.42857143 -0.41428571 -0.4 -0.38571429 -0.37142857 -0.35714286 -0.34285714 -0.32857143 -0.31428571 -0.3 -0.28571429 -0.27142857 -0.25714286 -0.24285714 -0.22857143 -0.21428571 -0.2 -0.18571429 -0.17142857 -0.15714286 -0.14285714 -0.12857143 -0.11428571 -0.1 -0.08571429 -0.07142857 -0.05714286 -0.04285714 -0.02857143 -0.01428571 0 0 0 0 0 0
  line L13 (-93.8265, 11.3727) -> (-93.8649, 11.8584)
  arc A27 (-93.7741, 11.9659) -> (-93.8649, 11.8584) centre (-93.7653, 11.8663) ccw
  arc A28 (-93.7741, 11.9659) -> (-92.7597, 12.0994) centre (-94.8448, 24.0176) ccw
  arc A29 (-92.6441, 12.0191) -> (-92.7597, 12.0994) centre (-92.7425, 12.0009) ccw
  line L14 (-92.6441, 12.0191) -> (-92.5556, 11.54)
  spline S14 degree 5 poles (-92.5556, 11.54) (-92.5545, 11.5344) (-92.5524, 11.5233) (-92.5487, 11.5068) (-92.543, 11.4849) (-92.5348, 11.4578) (-92.5258, 11.4309) (-92.5164, 11.4041) (-92.5067, 11.3773) (-92.4967, 11.3506) (-92.4866, 11.3239) (-92.4763, 11.2972) (-92.4657, 11.2706) (-92.4546, 11.2442) (-92.4432, 11.2178) (-92.4315, 11.1915) (-92.4195, 11.1653) (-92.4072, 11.1391) (-92.3946, 11.1131) (-92.3819, 11.087) (-92.369, 11.061) (-92.3558, 11.0351) (-92.3425, 11.0093) (-92.3289, 10.9835) (-92.315, 10.9577) (-92.301, 10.9321) (-92.2867, 10.9065) (-92.2723, 10.8809) (-92.2576, 10.8555) (-92.2428, 10.83) (-92.2277, 10.8047) (-92.2125, 10.7794) (-92.1971, 10.7541) (-92.1815, 10.7289) (-92.1657, 10.7038) (-92.1498, 10.6787) (-92.1337, 10.6537) (-92.1174, 10.6288) (-92.1009, 10.6039) (-92.0842, 10.579) (-92.0674, 10.5542) (-92.0504, 10.5295) (-92.0333, 10.5048) (-92.016, 10.4802) (-91.9985, 10.4557) (-91.9809, 10.4312) (-91.9631, 10.4068) (-91.9452, 10.3824) (-91.9271, 10.3581) (-91.9089, 10.3338) (-91.8905, 10.3096) (-91.8719, 10.2855) (-91.8532, 10.2614) (-91.8344, 10.2374) (-91.8154, 10.2134) (-91.7963, 10.1895) (-91.777, 10.1656) (-91.7576, 10.1418) (-91.738, 10.1181) (-91.7183, 10.0944) (-91.6984, 10.0708) (-91.6785, 10.0473) (-91.6583, 10.0238) (-91.6381, 10.0003) (-91.6177, 9.977) (-91.5972, 9.9536) (-91.5765, 9.9304) (-91.5557, 9.9072) (-91.5348, 9.8841) (-91.5137, 9.861) (-91.4925, 9.838) (-91.4754, 9.8196) (-91.4626, 9.8059) (-91.454, 9.7967) (-91.4497, 9.7921) knots 0 0 0 0 0 0 0.01428571 0.02857143 0.04285714 0.05714286 0.07142857 0.08571429 0.1 0.11428571 0.12857143 0.14285714 0.15714286 0.17142857 0.18571429 0.2 0.21428571 0.22857143 0.24285714 0.25714286 0.27142857 0.28571429 0.3 0.31428571 0.32857143 0.34285714 0.35714286 0.37142857 0.38571429 0.4 0.41428571 0.42857143 0.44285714 0.45714286 0.47142857 0.48571429 0.5 0.51428571 0.52857143 0.54285714 0.55714286 0.57142857 0.58571429 0.6 0.61428571 0.62857143 0.64285714 0.65714286 0.67142857 0.68571429 0.7 0.71428571 0.72857143 0.74285714 0.75714286 0.77142857 0.78571429 0.8 0.81428571 0.82857143 0.84285714 0.85714286 0.87142857 0.88571429 0.9 0.91428571 0.92857143 0.94285714 0.95714286 0.97142857 0.98571429 1 1 1 1 1 1
  arc A30 (-91.4497, 9.7921) -> (-90.6722, 10.0004) centre (-94.8448, 24.0176) ccw
  spline S15 degree 5 poles (-90.6722, 10.0004) (-90.6708, 10.0066) (-90.6679, 10.0188) (-90.6637, 10.0371) (-90.6581, 10.0615) (-90.6512, 10.0921) (-90.6445, 10.1226) (-90.638, 10.1531) (-90.6315, 10.1836) (-90.6253, 10.2141) (-90.6191, 10.2445) (-90.6132, 10.275) (-90.6073, 10.3054) (-90.6017, 10.3358) (-90.5961, 10.3662) (-90.5908, 10.3966) (-90.5855, 10.4269) (-90.5805, 10.4572) (-90.5755, 10.4876) (-90.5708, 10.5178) (-90.5661, 10.5481) (-90.5617, 10.5784) (-90.5574, 10.6086) (-90.5532, 10.6388) (-90.5492, 10.669) (-90.5454, 10.6991) (-90.5417, 10.7293) (-90.5382, 10.7594) (-90.5349, 10.7895) (-90.5317, 10.8195) (-90.5287, 10.8495) (-90.5258, 10.8795) (-90.5232, 10.9095) (-90.5206, 10.9394) (-90.5183, 10.9693) (-90.5161, 10.9992) (-90.5141, 11.029) (-90.5123, 11.0588) (-90.5107, 11.0886) (-90.5092, 11.1183) (-90.5079, 11.148) (-90.5068, 11.1776) (-90.5059, 11.2073) (-90.5052, 11.2368) (-90.5047, 11.2664) (-90.5044, 11.2958) (-90.5042, 11.3253) (-90.5043, 11.3547) (-90.5045, 11.384) (-90.5049, 11.4133) (-90.5056, 11.4426) (-90.5065, 11.4718) (-90.5076, 11.5009) (-90.509, 11.53) (-90.5105, 11.559) (-90.5123, 11.588) (-90.5143, 11.6169) (-90.5165, 11.6457) (-90.519, 11.6745) (-90.5216, 11.7032) (-90.5246, 11.7319) (-90.5279, 11.7604) (-90.5316, 11.7889) (-90.5357, 11.8172) (-90.5401, 11.8454) (-90.5447, 11.8736) (-90.5494, 11.9017) (-90.5544, 11.9298) (-90.5596, 11.9577) (-90.5654, 11.9855) (-90.5718, 12.0131) (-90.5778, 12.0349) (-90.5829, 12.0511) (-90.5865, 12.0618) (-90.5884, 12.0671) knots -1 -1 -1 -1 -1 -1 -0.98571429 -0.97142857 -0.95714286 -0.94285714 -0.92857143 -0.91428571 -0.9 -0.88571429 -0.87142857 -0.85714286 -0.84285714 -0.82857143 -0.81428571 -0.8 -0.78571429 -0.77142857 -0.75714286 -0.74285714 -0.72857143 -0.71428571 -0.7 -0.68571429 -0.67142857 -0.65714286 -0.64285714 -0.62857143 -0.61428571 -0.6 -0.58571429 -0.57142857 -0.55714286 -0.54285714 -0.52857143 -0.51428571 -0.5 -0.48571429 -0.47142857 -0.45714286 -0.44285714 -0.42857143 -0.41428571 -0.4 -0.38571429 -0.37142857 -0.35714286 -0.34285714 -0.32857143 -0.31428571 -0.3 -0.28571429 -0.27142857 -0.25714286 -0.24285714 -0.22857143 -0.21428571 -0.2 -0.18571429 -0.17142857 -0.15714286 -0.14285714 -0.12857143 -0.11428571 -0.1 -0.08571429 -0.07142857 -0.05714286 -0.04285714 -0.02857143 -0.01428571 0 0 0 0 0 0
  line L15 (-90.5884, 12.0671) -> (-90.7513, 12.5263)
  arc A31 (-90.6914, 12.6536) -> (-90.7513, 12.5263) centre (-90.657, 12.5597) ccw
  arc A32 (-90.6914, 12.6536) -> (-89.7461, 13.0452) centre (-94.8448, 24.0176) ccw
  arc A33 (-89.6137, 12.9975) -> (-89.7461, 13.0452) centre (-89.704, 12.9545) ccw
  line L16 (-89.6137, 12.9975) -> (-89.4041, 12.5577)
  spline S16 degree 5 poles (-89.4041, 12.5577) (-89.4017, 12.5525) (-89.3967, 12.5424) (-89.3889, 12.5274) (-89.3777, 12.5077) (-89.3628, 12.4836) (-89.3472, 12.4599) (-89.3311, 12.4365) (-89.3148, 12.4131) (-89.2983, 12.3899) (-89.2816, 12.3667) (-89.2647, 12.3436) (-89.2476, 12.3207) (-89.2301, 12.298) (-89.2122, 12.2755) (-89.1941, 12.2531) (-89.1757, 12.2309) (-89.157, 12.2089) (-89.1382, 12.1869) (-89.1192, 12.165) (-89.0999, 12.1433) (-89.0805, 12.1217) (-89.0609, 12.1001) (-89.0411, 12.0788) (-89.0211, 12.0575) (-89.0009, 12.0363) (-88.9805, 12.0153) (-88.9599, 11.9944) (-88.9391, 11.9735) (-88.9182, 11.9528) (-88.8971, 11.9322) (-88.8759, 11.9117) (-88.8545, 11.8913) (-88.8329, 11.871) (-88.8112, 11.8508) (-88.7893, 11.8307) (-88.7672, 11.8108) (-88.745, 11.7909) (-88.7226, 11.7711) (-88.7001, 11.7514) (-88.6775, 11.7318) (-88.6547, 11.7123) (-88.6317, 11.6929) (-88.6087, 11.6736) (-88.5854, 11.6545) (-88.5621, 11.6354) (-88.5386, 11.6164) (-88.5149, 11.5975) (-88.4912, 11.5786) (-88.4673, 11.5599) (-88.4432, 11.5413) (-88.4191, 11.5228) (-88.3948, 11.5044) (-88.3704, 11.486) (-88.3458, 11.4678) (-88.3212, 11.4497) (-88.2964, 11.4316) (-88.2714, 11.4137) (-88.2464, 11.3958) (-88.2212, 11.378) (-88.196, 11.3604) (-88.1706, 11.3428) (-88.145, 11.3253) (-88.1194, 11.3079) (-88.0937, 11.2906) (-88.0678, 11.2734) (-88.0418, 11.2563) (-88.0157, 11.2393) (-87.9895, 11.2223) (-87.9632, 11.2055) (-87.9368, 11.1887) (-87.9155, 11.1754) (-87.8996, 11.1655) (-87.8889, 11.1589) (-87.8835, 11.1556) knots 0 0 0 0 0 0 0.01428571 0.02857143 0.04285714 0.05714286 0.07142857 0.08571429 0.1 0.11428571 0.12857143 0.14285714 0.15714286 0.17142857 0.18571429 0.2 0.21428571 0.22857143 0.24285714 0.25714286 0.27142857 0.28571429 0.3 0.31428571 0.32857143 0.34285714 0.35714286 0.37142857 0.38571429 0.4 0.41428571 0.42857143 0.44285714 0.45714286 0.47142857 0.48571429 0.5 0.51428571 0.52857143 0.54285714 0.55714286 0.57142857 0.58571429 0.6 0.61428571 0.62857143 0.64285714 0.65714286 0.67142857 0.68571429 0.7 0.71428571 0.72857143 0.74285714 0.75714286 0.77142857 0.78571429 0.8 0.81428571 0.82857143 0.84285714 0.85714286 0.87142857 0.88571429 0.9 0.91428571 0.92857143 0.94285714 0.95714286 0.97142857 0.98571429 1 1 1 1 1 1
  arc A34 (-87.8835, 11.1556) -> (-87.1865, 11.558) centre (-94.8448, 24.0176) ccw
  spline S17 degree 5 poles (-87.1865, 11.558) (-87.1867, 11.5643) (-87.1871, 11.5768) (-87.1877, 11.5956) (-87.1886, 11.6207) (-87.1899, 11.6519) (-87.1913, 11.6832) (-87.1929, 11.7143) (-87.1946, 11.7454) (-87.1964, 11.7765) (-87.1984, 11.8075) (-87.2005, 11.8384) (-87.2027, 11.8693) (-87.2051, 11.9002) (-87.2077, 11.931) (-87.2103, 11.9617) (-87.2131, 11.9924) (-87.2161, 12.023) (-87.2192, 12.0535) (-87.2224, 12.084) (-87.2258, 12.1145) (-87.2293, 12.1448) (-87.233, 12.1752) (-87.2368, 12.2054) (-87.2407, 12.2356) (-87.2448, 12.2657) (-87.2491, 12.2958) (-87.2535, 12.3258) (-87.258, 12.3557) (-87.2627, 12.3855) (-87.2676, 12.4153) (-87.2726, 12.445) (-87.2778, 12.4746) (-87.2831, 12.5042) (-87.2886, 12.5337) (-87.2942, 12.5631) (-87.3, 12.5924) (-87.306, 12.6217) (-87.3121, 12.6509) (-87.3184, 12.68) (-87.3248, 12.709) (-87.3314, 12.7379) (-87.3382, 12.7667) (-87.3452, 12.7955) (-87.3523, 12.8241) (-87.3596, 12.8527) (-87.3671, 12.8812) (-87.3747, 12.9096) (-87.3826, 12.9378) (-87.3906, 12.966) (-87.3988, 12.9941) (-87.4072, 13.0221) (-87.4158, 13.0499) (-87.4247, 13.0777) (-87.4337, 13.1053) (-87.4429, 13.1328) (-87.4523, 13.1602) (-87.4619, 13.1875) (-87.4717, 13.2147) (-87.4818, 13.2418) (-87.492, 13.2686) (-87.5026, 13.2954) (-87.5136, 13.3219) (-87.5248, 13.3482) (-87.5363, 13.3743) (-87.5481, 13.4004) (-87.56, 13.4263) (-87.572, 13.4521) (-87.5843, 13.4777) (-87.597, 13.5031) (-87.6104, 13.528) (-87.6219, 13.5475) (-87.6309, 13.5619) (-87.6372, 13.5713) (-87.6404, 13.5759) knots -1 -1 -1 -1 -1 -1 -0.98571429 -0.97142857 -0.95714286 -0.94285714 -0.92857143 -0.91428571 -0.9 -0.88571429 -0.87142857 -0.85714286 -0.84285714 -0.82857143 -0.81428571 -0.8 -0.78571429 -0.77142857 -0.75714286 -0.74285714 -0.72857143 -0.71428571 -0.7 -0.68571429 -0.67142857 -0.65714286 -0.64285714 -0.62857143 -0.61428571 -0.6 -0.58571429 -0.57142857 -0.55714286 -0.54285714 -0.52857143 -0.51428571 -0.5 -0.48571429 -0.47142857 -0.45714286 -0.44285714 -0.42857143 -0.41428571 -0.4 -0.38571429 -0.37142857 -0.35714286 -0.34285714 -0.32857143 -0.31428571 -0.3 -0.28571429 -0.27142857 -0.25714286 -0.24285714 -0.22857143 -0.21428571 -0.2 -0.18571429 -0.17142857 -0.15714286 -0.14285714 -0.12857143 -0.11428571 -0.1 -0.08571429 -0.07142857 -0.05714286 -0.04285714 -0.02857143 -0.01428571 0 0 0 0 0 0
  line L17 (-87.6404, 13.5759) -> (-87.9166, 13.9773)
  arc A35 (-87.8917, 14.1158) -> (-87.9166, 13.9773) centre (-87.8342, 14.034) ccw
  arc A36 (-87.8917, 14.1158) -> (-87.08, 14.7387) centre (-94.8448, 24.0176) ccw
  arc A37 (-86.9397, 14.7269) -> (-87.08, 14.7387) centre (-87.0158, 14.662) ccw
  line L18 (-86.9397, 14.7269) -> (-86.6235, 14.3563)
  spline S18 degree 5 poles (-86.6235, 14.3563) (-86.6198, 14.352) (-86.6123, 14.3435) (-86.6009, 14.331) (-86.585, 14.3149) (-86.5644, 14.2955) (-86.5431, 14.2767) (-86.5215, 14.2581) (-86.4997, 14.2398) (-86.4778, 14.2216) (-86.4557, 14.2035) (-86.4334, 14.1856) (-86.4109, 14.168) (-86.3881, 14.1505) (-86.3651, 14.1334) (-86.3418, 14.1165) (-86.3182, 14.0998) (-86.2945, 14.0833) (-86.2706, 14.067) (-86.2466, 14.0508) (-86.2224, 14.0348) (-86.1981, 14.0189) (-86.1735, 14.0032) (-86.1489, 13.9876) (-86.124, 13.9723) (-86.099, 13.9571) (-86.0739, 13.942) (-86.0486, 13.9272) (-86.0231, 13.9124) (-85.9976, 13.8978) (-85.9719, 13.8834) (-85.946, 13.8691) (-85.9201, 13.8549) (-85.894, 13.8409) (-85.8678, 13.827) (-85.8414, 13.8133) (-85.8149, 13.7997) (-85.7883, 13.7862) (-85.7616, 13.7729) (-85.7348, 13.7597) (-85.7078, 13.7466) (-85.6808, 13.7337) (-85.6536, 13.7209) (-85.6263, 13.7083) (-85.5989, 13.6957) (-85.5714, 13.6833) (-85.5438, 13.6711) (-85.5161, 13.6589) (-85.4882, 13.6469) (-85.4603, 13.635) (-85.4323, 13.6233) (-85.4041, 13.6116) (-85.3759, 13.6001) (-85.3476, 13.5887) (-85.3191, 13.5775) (-85.2906, 13.5663) (-85.262, 13.5553) (-85.2333, 13.5444) (-85.2045, 13.5337) (-85.1756, 13.523) (-85.1466, 13.5125) (-85.1175, 13.5021) (-85.0883, 13.4918) (-85.0591, 13.4816) (-85.0297, 13.4716) (-85.0003, 13.4617) (-84.9707, 13.4518) (-84.9411, 13.4422) (-84.9114, 13.4326) (-84.8817, 13.4231) (-84.8518, 13.4138) (-84.8278, 13.4064) (-84.8098, 13.4009) (-84.7978, 13.3973) (-84.7918, 13.3955) knots 0 0 0 0 0 0 0.01428571 0.02857143 0.04285714 0.05714286 0.07142857 0.08571429 0.1 0.11428571 0.12857143 0.14285714 0.15714286 0.17142857 0.18571429 0.2 0.21428571 0.22857143 0.24285714 0.25714286 0.27142857 0.28571429 0.3 0.31428571 0.32857143 0.34285714 0.35714286 0.37142857 0.38571429 0.4 0.41428571 0.42857143 0.44285714 0.45714286 0.47142857 0.48571429 0.5 0.51428571 0.52857143 0.54285714 0.55714286 0.57142857 0.58571429 0.6 0.61428571 0.62857143 0.64285714 0.65714286 0.67142857 0.68571429 0.7 0.71428571 0.72857143 0.74285714 0.75714286 0.77142857 0.78571429 0.8 0.81428571 0.82857143 0.84285714 0.85714286 0.87142857 0.88571429 0.9 0.91428571 0.92857143 0.94285714 0.95714286 0.97142857 0.98571429 1 1 1 1 1 1
  arc A38 (-84.7918, 13.3955) -> (-84.2227, 13.9647) centre (-94.8448, 24.0176) ccw